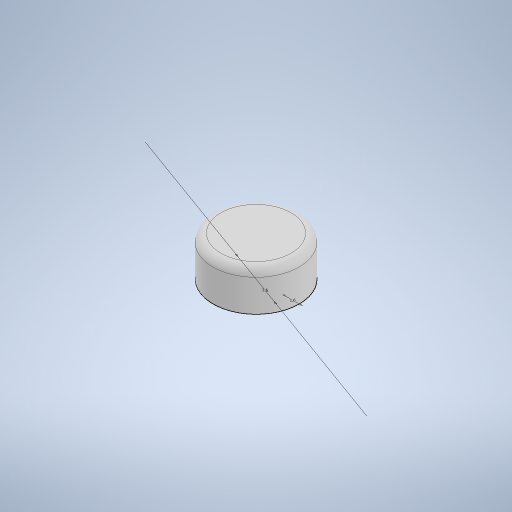
# Autodesk Inventor part: final_탄두낙하산거치대_스프링고정
Saved by Autodesk Inventor 2023 (Build 270158000, 158)
## iProperties
Created: 2023-11-22
Part Number: final_탄두낙하산거치대_스프링고정
Material: 일반
Document SubType Name: Modeling
Designer: rlatk
Density: 1 g/cm^3
Appearance: 기본값
Author: rlatk
Autodesk Inventor part; units mm, degrees
ref_plane "YZ Plane" through (0, 0, 0) normal (1, 0, 0) x (0, 1, 0)
ref_plane "XZ Plane" through (0, 0, 0) normal (0, 1, 0) x (-1, 0, 0)
ref_plane "XY Plane" through (0, 0, 0) normal (0, 0, 1) x (1, 0, 0)
sketch "스케치1" plane through (0, 0, 0) normal (0, 1, 0) x (-1, 0, 0)
  circle A0 centre (0, 0) radius 3.8
  circle A1 centre (0, 0) radius 5.4
  dimension "d0" = 7.6
  dimension "d1" = 1.6
  constraints: 2 centre point, 1 coincident
  measures "d0" diameter of A0
  measures "d1" radial gap between concentric circles of A0 A1
extrude "돌출1" add sketch "스케치1" along normal blind 5 contours A0 | A1
extrude "돌출2" cut sketch "스케치1" along normal blind 3.4 contours A0
fillet "모깎기1" radius 1 1 edges at (5.4, 5, 0)
